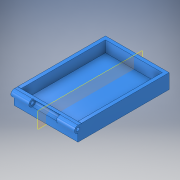
# Autodesk Inventor part: TopHalfOfBoard
Saved by Autodesk Inventor 2017 SP1 (Build 210196100, 196)
## iProperties
Created: 2016-10-19
Part Number: TopHalfOfBoard
Material: ABS Plastic
Document SubType Name: Modeling
Designer: steele
Density: 1.06 g/cm^3
Appearance: Cyan
Author: steele
Autodesk Inventor part; units mm, degrees
ref_plane "YZ Plane" through (0, 0, 0) normal (1, 0, 0) x (0, 1, 0)
ref_plane "XZ Plane" through (0, 0, 0) normal (0, 1, 0) x (-1, 0, 0)
ref_plane "XY Plane" through (0, 0, 0) normal (0, 0, 1) x (1, 0, 0)
sketch "Sketch2" plane through (0, 0, 0) normal (0, 1, 0) x (-1, 0, 0)
  line L0 (29.3687, 42.0688) -> (-29.3688, 42.0688)
  line L1 (-29.3688, 42.0688) -> (-29.3687, -42.0688)
  line L2 (-29.3687, -42.0688) -> (29.3688, -42.0688)
  line L3 (29.3688, -42.0688) -> (29.3687, 42.0688)
  line L4 (29.3687, 42.0688) -> (-29.3687, -42.0688) construction
  line L5 (-29.3688, 42.0688) -> (29.3688, -42.0688) construction
  point P0 (0, 0)
  dimension "d4" = 58.7375
  dimension "d5" = 84.1375
  constraints: 12 end point, 2 midpoint, 2 parallel, 1 horizontal, 1 perpendicular
  measures "d4" distance of L1.end L2.end
  measures "d5" distance of L2.end L0.start
extrude "Extrusion1" add sketch "Sketch2" against normal blind 3.175
sketch "Sketch3" plane through (0, 0, 0) normal (0, 1, 0) x (1, 0, 0)
  line L0 (29.3688, -42.0688) -> (-29.3687, -42.0688) projected
  line L1 (-29.3688, 42.0688) -> (29.3687, 42.0688) projected
  line L2 (-29.3687, -42.0688) -> (29.3687, -42.0688)
  line L3 (29.3687, -42.0688) -> (29.3687, 42.0688)
  line L4 (29.3687, 42.0688) -> (-29.3687, 42.0688)
  line L5 (-29.3687, 42.0688) -> (-29.3687, -42.0688)
  line L6 (-26.1938, -38.8937) -> (26.1937, -38.8937)
  line L7 (26.1937, -38.8937) -> (26.1937, 38.8937)
  line L8 (26.1937, 38.8937) -> (-26.1938, 38.8937)
  line L9 (-26.1938, 38.8937) -> (-26.1938, -38.8937)
  line L10 (-26.1938, -38.8937) -> (26.1937, 38.8937) construction
  line L11 (26.1937, -38.8937) -> (-26.1938, 38.8937) construction
  point P0 (0, 0)
  dimension "d8" = 3.175
  dimension "d9" = 3.175
  constraints: 20 end point, 4 parallel, 2 horizontal, 2 midpoint, 2 perpendicular
  measures "d8" distance between parallel lines of L6 L0
  measures "d9" distance between parallel lines of L3 L7
extrude "Extrusion2" add sketch "Sketch3" along normal blind 7.1437
sketch "Sketch6" plane through (-29.3688, -3.175, -42.0688) normal (-1, 0, 0) x (0, 0, 1)
  line L0 (0, 10.3187) -> (84.1375, 10.3187) projected
  line L1 (84.1375, 10.3187) -> (84.1375, 0) projected
  circle A0 centre (84.1375, 10.3187) radius 3.175
  point P0 (42.0688, 3.175)
  dimension "d16" = 6.35
  constraints: 1 centre point, 1 coincident
  measures "d16" diameter of A0
extrude "Extrusion5" add sketch "Sketch6" against normal blind 58.7375
sketch "Sketch8" plane through (-29.3688, -3.175, -42.0688) normal (-1, 0, 0) x (0, 0, 1)
  arc A0 (84.1375, 7.1437) -> (80.9625, 10.3187) centre (84.1375, 10.3187) ccw projected
  circle A1 centre (84.1375, 10.3187) radius 1.5875
  point P0 (42.0688, 3.175)
  dimension "d21" = 3.175
  constraints: 1 centre point, 1 coincident
  measures "d21" diameter of A1
extrude "Extrusion6" cut sketch "Sketch8" against normal blind 58.7375
sketch "Sketch11" plane through (0, 7.1437, 0) normal (0, 1, 0) x (1, 0, 0)
  line L0 (-29.3688, 42.0688) -> (29.3687, 42.0688) projected
  line L1 (-29.3688, 42.0688) -> (29.3687, 42.0688)
  line L2 (29.3687, 42.0688) -> (29.3688, -38.7648)
  line L3 (29.3687, 42.0688) -> (29.3688, -42.0688) projected
  line L4 (26.1937, -38.8937) -> (29.3688, -38.8937) projected
  line L5 (26.1937, 38.8937) -> (26.1937, -38.8937) projected
  line L6 (26.1937, -38.8937) -> (26.1937, 38.8937)
  line L7 (26.1937, 38.8937) -> (-26.1938, 38.8937)
  line L8 (-29.3687, -38.8938) -> (-26.1938, -38.8937) projected
  line L9 (-26.1938, 38.8937) -> (-26.1938, -38.8937)
  line L10 (-26.1938, -38.8937) -> (-29.3687, -38.8938)
  line L11 (-29.3688, 42.0688) -> (-29.3687, -38.8938) projected
  line L12 (-29.3687, -38.8938) -> (-29.3688, 42.0688)
  point P0 (0, 0)
  constraints: 14 end point, 2 collinear, 2 perpendicular, 1 horizontal, 1 parallel, 1 point on line
extrude "Extrusion9" add sketch "Sketch11" along normal blind 3.175
sketch "Sketch12" plane through (-29.3688, -3.175, -42.0688) normal (-1, 0, 0) x (0, 0, 1)
  line L0 (80.9625, 3.175) -> (80.9625, 10.3187) projected
  line L1 (80.9625, 10.3187) -> (80.9625, 13.3208)
  arc A0 (84.1375, 7.1437) -> (80.9625, 10.3187) centre (84.1375, 10.3187) ccw projected
  line L2 (80.9625, 13.3208) -> (83.9598, 13.4888)
  point P0 (42.0688, 3.175)
  constraints: 4 end point, 2 tangent, 1 point on circle, 1 vertical
extrude "Extrusion10" add sketch "Sketch12" against normal blind 58.7375
ref_plane "Work Plane1" through (-0.0063, -3.175, 42.0688) normal (1, 0, 0) x (0, 0, -1)
sketch "Sketch13" plane through (-0.0063, -3.175, 42.0688) normal (1, 0, 0) x (0, 0, -1)
  circle A0 centre (0, 10.3187) radius 1.5875 projected
  circle A1 centre (0, 10.3187) radius 3.175
  point P0 (42.0688, 3.175)
  dimension "d33" = 6.35
  constraints: 1 centre point, 1 coincident
  measures "d33" diameter of A1
extrude "Extrusion11" cut sketch "Sketch13" along normal mid plane 25.4
equation "\"d4\" = 2 * materialWallThickness + cardDeckWidth + cardDeckAirGap"
equation "\"d5\" = 2 * materialWallThickness + cardDeckLength + cardDeckAirGap"
equation "\"d6\" = baseWallThickness"
equation "\"d8\" = baseWallThickness"
equation "\"d9\" = baseWallThickness"
equation "\"d10\" = 0.5 * cardDeckDepth"
equation "\"d19\" = d4"
equation "\"d22\" = d4"
equation "\"d30\" = d4"
equation "\"cardDeckWidth\" = 50.8"
equation "\"cardDeckLength\" = 76.2"
equation "\"d0\" = cardDeckWidth"
equation "\"d1\" = cardDeckLength"
equation "\"cardDeckDepth\" = 14.2875"
equation "\"d2\" = cardDeckDepth"
equation "\"d3\" = 0"
equation "\"materialWallThickness\" = 3.175"
equation "\"baseWallThickness\" = 3.175"
equation "\"cardDeckAirGap\" = 1.5875"
equation "\"hingeOuterDiam\" = 12.7"
equation "\"hingeInnerDiam\" = 6.35"
body "Solid1"
